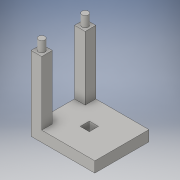
# Autodesk Inventor part: Maglev_top
Saved by Autodesk Inventor 2016 (Build 200138000, 138)
## iProperties
Created: 2018-01-06
Part Number: Maglev_top
Material: Generic
Document SubType Name: Modeling
Designer: Jorian Bruslind
Density: 1 g/cm^3
Appearance: Default
Author: Jorian Bruslind
Autodesk Inventor part; units mm, degrees
ref_plane "YZ Plane" through (0, 0, 0) normal (1, 0, 0) x (0, 1, 0)
ref_plane "XZ Plane" through (0, 0, 0) normal (0, 1, 0) x (-1, 0, 0)
ref_plane "XY Plane" through (0, 0, 0) normal (0, 0, 1) x (1, 0, 0)
sketch "Sketch1" plane through (0, 0, 0) normal (0, 1, 0) x (-1, 0, 0)
  line L0 (0, 0) -> (-76.2, 0)
  line L1 (-76.2, 0) -> (-76.2, -64.6684)
  line L2 (-76.2, -64.6684) -> (0, -64.6684)
  line L3 (0, -64.6684) -> (0, 0)
  line L4 (0, -32.3342) -> (-31.75, -32.3342)
  line L5 (-31.75, -32.3342) -> (-31.75, -37.8342)
  line L6 (-31.75, -37.8342) -> (-42.75, -37.8342)
  line L7 (-42.75, -37.8342) -> (-42.75, -26.8342)
  line L8 (-42.75, -26.8342) -> (-31.75, -26.8342)
  line L9 (-31.75, -26.8342) -> (-31.75, -37.8342)
  dimension "d0" = 76.2
  dimension "d1" = 64.6684
  dimension "d2" = 31.75
  dimension "d3" = 5.5
  dimension "d4" = 11
  dimension "d5" = 11
  constraints: 20 end point, 4 parallel, 3 horizontal, 2 perpendicular, 1 midpoint, 1 vertical
  measures "d0" distance of L2.end L1.end
  measures "d1" distance of L1.end L0.end
  measures "d2" distance of L4.start L4.end
  measures "d3" distance of L4.end L5.end
  measures "d4" distance of L7.end L8.end
  measures "d5" distance of L6.end L7.end
extrude "Extrusion1" add sketch "Sketch1" along normal blind 12.7
sketch "Sketch2" plane through (0, 12.7, 0) normal (0, 1, 0) x (1, 0, 0)
  line L0 (0, 0) -> (76.2, 0) projected
  line L1 (0, 0) -> (12.7, 0)
  line L2 (12.7, 0) -> (12.7, 12.7)
  line L3 (12.7, 12.7) -> (0, 12.7)
  line L4 (0, 12.7) -> (0, 0)
  line L5 (0, 64.6684) -> (12.7, 64.6684)
  line L6 (12.7, 64.6684) -> (12.7, 51.9684)
  line L7 (12.7, 51.9684) -> (0, 51.9684)
  line L8 (0, 51.9684) -> (0, 64.6684)
  dimension "d8" = 12.7
  dimension "d9" = 12.7
  dimension "d10" = 12.7
  dimension "d11" = 12.7
  constraints: 16 end point, 4 parallel, 2 horizontal, 2 perpendicular
  measures "d8" distance of L3.end L2.end
  measures "d9" distance of L2.end L1.end
  measures "d10" distance of L6.end L7.end
  measures "d11" distance of L5.end L6.end
extrude "Extrusion2" add sketch "Sketch2" along normal blind 76.2
sketch "Sketch3" plane through (0, 88.9, 0) normal (0, 1, 0) x (1, 0, 0)
  line L0 (0, 0) -> (0, 6.35)
  line L1 (0, 64.6684) -> (0, 0) projected
  line L2 (0, 6.35) -> (6.35, 6.35)
  circle A0 centre (6.35, 6.35) radius 3.81
  line L3 (0, 64.6684) -> (0, 58.3184)
  line L4 (0, 58.3184) -> (6.35, 58.3184)
  circle A1 centre (6.35, 58.3184) radius 3.81
  dimension "d14" = 6.35
  dimension "d15" = 6.35
  dimension "d16" = 7.62
  dimension "d17" = 6.35
  dimension "d18" = 7.62
  constraints: 8 end point, 2 centre point, 2 coincident, 2 perpendicular, 2 point on line
  measures "d14" distance of L0.start L0.end
  measures "d15" distance of L0.end L2.end
  measures "d16" diameter of A0
  measures "d17" distance of L1.start L3.end
  measures "d18" diameter of A1
extrude "Extrusion3" add sketch "Sketch3" along normal blind 12.7
body "Solid1"
